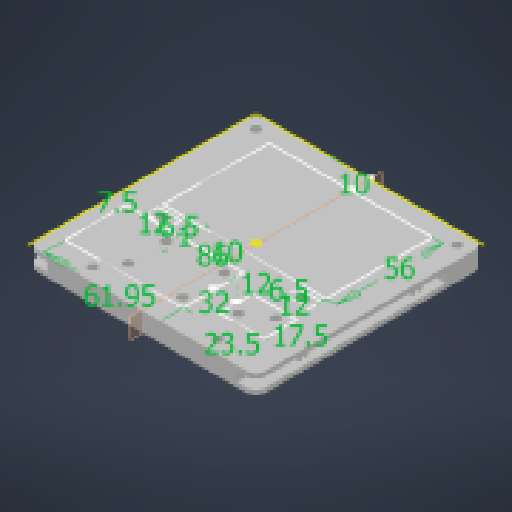
# Autodesk Inventor part: PCB_Housing_01_003
Saved by Autodesk Inventor 2026.2 (Build 302298000, 298)
## iProperties
Created: 2026-02-18
Part Number: PCB_Housing_01_003
Material: Generic
Document SubType Name: Modeling
Designer: vckot
Density: 1 g/cm^3
Appearance: Default
Author: vckot
Autodesk Inventor part; units mm, degrees
ref_plane "YZ Plane" through (0, 0, 0) normal (1, 0, 0) x (0, 1, 0)
ref_plane "XZ Plane" through (0, 0, 0) normal (0, 1, 0) x (-1, 0, 0)
ref_plane "XY Plane" through (0, 0, 0) normal (0, 0, 1) x (1, 0, 0)
sketch "Sketch1" plane through (0, 0, 0) normal (0, 1, 0) x (-1, 0, 0)
  line L0 (-60, 60) -> (60, 60)
  line L1 (60, 60) -> (60, -60)
  line L2 (60, -60) -> (-60, -60)
  line L3 (-60, -60) -> (-60, 60)
  line L4 (-60, 60) -> (60, -60) construction
  line L5 (60, 60) -> (-60, -60) construction
  point P0 (0, 0)
  dimension "d2" = 120
  dimension "d3" = 120
  constraints: 12 end point, 2 midpoint, 2 parallel, 1 horizontal, 1 perpendicular
  measures "d2" distance of L1.end L2.end
  measures "d3" distance of L0.end L1.end
extrude "Extrusion1" add sketch "Sketch1" along normal blind 10
sketch "Sketch2" plane through (0, 10, 0) normal (0, 1, 0) x (1, 0, 0)
  line L0 (-50, -43) -> (6, -43)
  line L1 (6, -43) -> (6, 43)
  line L2 (6, 43) -> (-50, 43)
  line L3 (-50, 43) -> (-50, -43)
  line L4 (-60, 60) -> (-60, -60) projected
  line L5 (-60, -60) -> (60, -60) projected
  line L6 (16, -52.5) -> (48, -52.5)
  line L7 (48, -52.5) -> (48, 9.45)
  line L8 (48, 9.45) -> (16, 9.45)
  line L9 (16, 9.45) -> (16, -52.5)
  line L10 (23.25, 21.45) -> (40.75, 21.45)
  line L11 (40.75, 21.45) -> (40.75, 44.95)
  line L12 (40.75, 44.95) -> (23.25, 44.95)
  line L13 (23.25, 44.95) -> (23.25, 21.45)
  line L14 (8.5, -43) -> (15, -43)
  line L15 (15, -43) -> (15, -31)
  line L16 (15, -31) -> (8.5, -31)
  line L17 (8.5, -31) -> (8.5, -43)
  line L18 (8.5, 43) -> (15, 43)
  line L19 (15, 43) -> (15, 31)
  line L20 (15, 31) -> (8.5, 31)
  line L21 (8.5, 31) -> (8.5, 43)
  point P0 (0, 0)
  point P1 (32, 21.45)
  point P2 (32, 9.45)
  point P3 (-50, 0)
  point P4 (-60, 0)
  dimension "d4" = 86
  dimension "d5" = 56
  dimension "d6" = 10
  dimension "d8" = 61.95
  dimension "d9" = 32
  dimension "d10" = 10
  dimension "d11" = 7.5
  dimension "d12" = 23.5
  dimension "d13" = 17.5
  dimension "d14" = 12
  dimension "d40" = 6.5
  dimension "d41" = 12
  dimension "d42" = 6.5
  dimension "d43" = 12
  dimension "d44" = 1
  constraints: 40 end point, 10 parallel, 5 horizontal, 5 perpendicular, 4 midpoint, 3 collinear, 1 horizontal alignment, 1 vertical alignment
  measures "d4" distance of L0.end L1.end
  measures "d5" distance of L1.end L2.end
  measures "d6" distance between parallel lines of L3 L4
  measures "d8" distance of L6.end L7.end
  measures "d9" distance of L7.end L8.end
  measures "d10" distance between parallel lines of L1 L9
  measures "d11" distance between parallel lines of L5 L6
  measures "d12" distance of L10.end L11.end
  measures "d13" distance of L11.end L12.end
  measures "d14" distance between parallel lines of L10 L8
  measures "d40" distance of L16.end L15.end
  measures "d41" distance of L15.end L14.end
  measures "d42" distance of L19.end L20.end
  measures "d43" distance of L18.end L19.end
  measures "d44" distance between parallel lines of L9 L15
fillet "Fillet1" radius 5 4 edges at (60, 5, -60) (60, 5, 60) (-60, 5, -60) (-60, 5, 60)
sketch "Sketch3" plane through (0, 0, 0) normal (0, -1, 0) x (1, 0, 0)
  circle A0 centre (22, 25.35) radius 2.675 projected
  circle A1 centre (42, 25.35) radius 2.675 projected
  circle A2 centre (28.25, -38.7) radius 2.675 projected
  circle A3 centre (35.75, -26.45) radius 2.675 projected
  circle A4 centre (43, -4.45) radius 2.675 projected
  circle A5 centre (21, -4.45) radius 2.675 projected
  circle A6 centre (53, 33) radius 2.675 projected
  circle A7 centre (53, -33) radius 2.675 projected
  circle A8 centre (-53, 53) radius 2.675 projected
  circle A9 centre (-53, -53) radius 2.675 projected
  circle A10 centre (11.75, 37) radius 2.675 projected
  circle A11 centre (11.75, -37) radius 2.675 projected
  point P0 (0, 0)
hole "Hole1" at (42, 0, 25.35) at (43, 0, -4.45) at (35.75, 0, -26.45) at (28.25, 0, -38.7) at (21, 0, -4.45) at (22, 0, 25.35) at (53, 0, 33) at (-53, 0, 53) at (-53, 0, -53) at (53, 0, -33) at (11.75, 0, 37) at (11.75, 0, -37) direction (0, 1, 0) diameter 4.7 end through all counterbore diameter 9 counterbore depth 4
sketch "Sketch4" plane through (55, 0, -60) normal (0, 0, -1) x (-1, 0, 0)
  line L0 (-5, 10) -> (-5, 0) projected
  line L1 (-5, 7.5) -> (95, 7.5)
  line L2 (95, 7.5) -> (95, 2.5)
  line L3 (95, 2.5) -> (-5, 2.5)
  line L4 (-5, 2.5) -> (-5, 7.5)
  point P0 (55, 0)
  point P1 (-5, 5)
  point P2 (-5, 5)
  point P3 (-5, 2.5)
  dimension "d23" = 5
  dimension "d24" = 100
  constraints: 8 end point, 2 midpoint, 2 parallel, 1 coincident, 1 horizontal, 1 perpendicular, 1 point on line
  measures "d23" distance between parallel lines of L3 L1
  measures "d24" distance between parallel lines of L2 L0
extrude "Extrusion2" cut sketch "Sketch4" against normal blind 10
sketch "Sketch5" plane through (-40, 7.5, -60) normal (0, -1, 0) x (1, 0, 0)
  arc A0 (17.5, 3) -> (12.5, 3) centre (15, 3) ccw
  line L0 (17.5, 3) -> (17.5, 0)
  line L1 (12.5, 3) -> (12.5, 0)
  line L2 (14, 0) -> (14, 3)
  arc A1 (16, 3) -> (14, 3) centre (15, 3) ccw
  line L3 (16, 3) -> (16, 0)
  line L4 (17.5, 0) -> (16, 0)
  line L5 (95, 0) -> (0, 0) projected
  line L6 (14, 0) -> (12.5, 0)
  line L7 (100, 10) -> (100, 5) projected
  point P0 (40, 60)
  dimension "d27" = 5
  dimension "d31" = 1.5
  dimension "d34" = 3
  dimension "d35" = 85
  dimension "d36" = 5
  constraints: 12 end point, 4 collinear, 4 point on circle, 2 centre point, 2 parallel, 1 tangent, 1 vertical, 2 other
  measures "d27" diameter of A0
  measures "d31" radial gap between concentric circles of A0 A1
  measures "d34" distance from line of L4 A0.centre
  measures "d35" distance from line of L7 A0.centre
  measures "d36" distance between parallel lines of L1 L0
extrude "Extrusion3" add sketch "Sketch5" along normal blind 2 contours L0 L4 L3 A1 L2 L5 L1 A0
pattern_linear "Rectangular Pattern1" count 2 spacing 60 along (1, 0, 0) of "Extrusion3"
ref_plane "Work Plane1" through (55, 0, 0) normal (0, 0, -1) x (-1, 0, 0)
mirror "Mirror1" about plane through (55, 0, 0) normal (0, 0, -1) of "Extrusion2", "Extrusion3", "Rectangular Pattern1"
body "Solid1"
